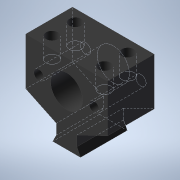
# Autodesk Inventor part: Slider
Saved by Autodesk Inventor 2021 (Build 250183000, 183)
## iProperties
Created: 2024-02-18
Part Number: Slider
Material: Generic
Document SubType Name: Modeling
Designer: Lukas
Density: 1 g/cm^3
Appearance: Default
Author: Lukas
Autodesk Inventor part; units mm, degrees
ref_plane "YZ Plane" through (0, 0, 0) normal (1, 0, 0) x (0, 1, 0)
ref_plane "XZ Plane" through (0, 0, 0) normal (0, 1, 0) x (-1, 0, 0)
ref_plane "XY Plane" through (0, 0, 0) normal (0, 0, 1) x (1, 0, 0)
sketch "Sketch1" plane through (0, 0, 0) normal (0, 0, 1) x (1, 0, 0)
  line L0 (-3.5, -11.25) -> (-3.5, -14.7505)
  line L1 (-3.5, -14.7505) -> (-4.75, -17.25)
  line L2 (-4.75, -17.25) -> (4.75, -17.25)
  line L3 (4.75, -17.25) -> (3.5, -14.7505)
  line L4 (3.5, -14.7505) -> (3.5, -11.25)
  line L5 (3.5, -11.25) -> (14, -6.25)
  line L6 (14, -6.25) -> (14, 10)
  line L7 (14, 10) -> (-14, 10)
  line L8 (-14, 10) -> (-14, -6.25)
  line L9 (-14, -6.25) -> (-3.5, -11.25)
  circle A0 centre (0, 0) radius 5.5
  circle A1 centre (-9.5, 0) radius 1.75
  circle A2 centre (9.5, 0) radius 1.75
  point P0 (0, 10)
  point P1 (0, -17.25)
  dimension "d0" = 11
  dimension "d1" = 17.25
  dimension "d2" = 7
  dimension "d3" = 9.5
  dimension "d4" = 63.43
  dimension "d5" = 6
  dimension "d6" = 5
  dimension "d7" = 28
  dimension "d8" = 3.5
  dimension "d9" = 19
  dimension "d10" = 9.5
  dimension "d11" = 10
  constraints: 20 end point, 4 horizontal alignment, 3 centre point, 3 perpendicular, 2 coincident, 2 equal length, 2 midpoint, 2 parallel, 2 vertical alignment, 1 equal radius, 1 vertical
  measures "d0" diameter of A0
  measures "d1" distance from line of L2 A0.centre
  measures "d2" distance between parallel lines of L4 L0
  measures "d3" distance of L1.end L2.end
  measures "d4" angle of L2 L1
  measures "d5" distance from line of L0.start L2
  measures "d6" vertical distance of L8.end L0.start
  measures "d7" distance of L6.end L7.end
  measures "d8" diameter of A2
  measures "d9" distance of A1.centre A2.centre
  measures "d10" distance of A1.centre point (0, 0)
  measures "d11" distance from line of L7 point (0, 0)
extrude "Extrusion1" add sketch "Sketch1" along normal blind 16
sketch "Sketch2" plane through (-14, 10, 0) normal (0, 1, 0) x (1, 0, 0)
  circle A0 centre (5, -4) radius 2.1
  circle A1 centre (5, -12) radius 2.1
  circle A2 centre (23, -12) radius 2.1
  circle A3 centre (23, -4) radius 2.1
  line L0 (28, 0) -> (0, 0) projected
  line L1 (28, -16) -> (0, -16) projected
  point P0 (14, 0)
  dimension "d14" = 18
  dimension "d15" = 9
  dimension "d17" = 4
  dimension "d18" = 4.2
  dimension "d19" = 4
  constraints: 4 centre point, 3 equal radius, 2 horizontal alignment, 2 vertical alignment
  measures "d14" distance of A3.centre A0.centre
  measures "d15" horizontal distance of point (14, 0) A0.centre
  measures "d17" distance from line of L0 A0.centre
  measures "d18" diameter of A0
  measures "d19" distance from line of L1 A1.centre
extrude "Extrusion2" cut sketch "Sketch2" against normal blind 7
equation "\"d10\" = 0.5 * d9"
equation "\"d15\" = 0.5 * d14"
equation "\"d19\" = d17"
body "Solid1"
